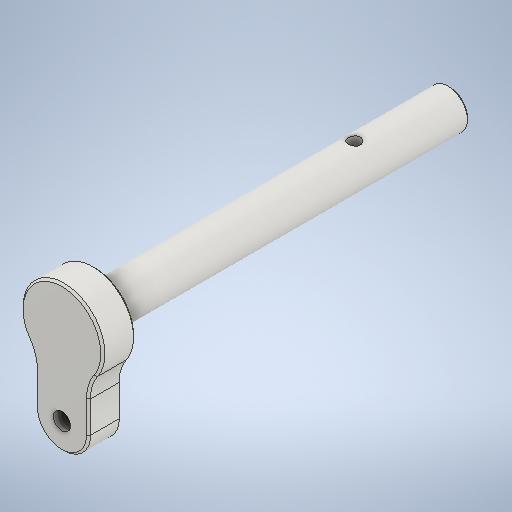
# Autodesk Inventor part: Crankshaft
Saved by Autodesk Inventor 2025.2 (Build 292293000, 293)
## iProperties
Created: 2025-06-12
Part Number: Crankshaft
Material: Steel AISI 1020 107 HR
Document SubType Name: Modeling
Designer: bless
Density: 7.87 g/cm^3
Appearance: Steel
Author: bless
Autodesk Inventor part; units mm, degrees
ref_plane "YZ Plane" through (0, 0, 0) normal (1, 0, 0) x (0, 1, 0)
ref_plane "XY Plane" through (0, 0, 0) normal (0, 0, 1) x (1, 0, 0)
sketch "Sketch1" plane through (0, 0, 0) normal (0, 0, 1) x (1, 0, 0)
  arc A0 (8.2491, -5.6527) -> (-8.2509, -5.65) centre (0, 0) ccw
  arc A1 (-6.5018, -19) -> (6.4982, -19) centre (-0.0018, -19) ccw
  circle A2 centre (0, 0) radius 4.75
  line L0 (-6.5018, -19) -> (-6.5018, -11.3)
  line L1 (6.4982, -19) -> (6.4982, -11.3053)
  arc A3 (-6.5018, -11.3) -> (-8.2509, -5.65) centre (-16.5018, -11.3) ccw
  arc A4 (8.2491, -5.6527) -> (6.4982, -11.3053) centre (16.4982, -11.3053) ccw
  point P0 (-6.5018, -7.5978)
  point P1 (6.4982, -7.6009)
  point P2 (-6.9491, -8.3427)
  dimension "d0" = 20
  dimension "d1" = 9.5
  dimension "d2" = 13
  dimension "d3" = 19
  dimension "d4" = 10
  dimension "d6" = 7.7
  constraints: 11 point on circle, 6 tangent, 5 centre point, 4 end point, 2 coincident, 2 point on line, 1 equal radius, 1 parallel, 1 vertical
  measures "d0" diameter of A0
  measures "d1" diameter of A2
  measures "d2" diameter of A1
  measures "d3" distance of A1.centre point (0, 0)
  measures "d4" radius of A3
  measures "d6" vertical distance of L0.end A1.centre
extrude "Extrusion1" add sketch "Sketch1" along normal blind 8
sketch "Sketch2" plane through (0, 0, 8) normal (0, 0, 1) x (1, 0, 0)
  arc A0 (-6.5018, -19) -> (6.4982, -19) centre (-0.0018, -19) ccw projected
hole "Hole1" at (-0.0018, -19, 8) direction (0, 0, -1) diameter 4.134 end through all thread size "M5x0.8" class "6H" standard "ANSI Metric M Profile"
sketch "Sketch3" plane through (0, 0, 8) normal (0, 0, 1) x (1, 0, 0)
  circle A0 centre (0, 0) radius 4.75 projected
  circle A1 centre (0, 0) radius 4.75
  constraints: 1 centre point, 1 coincident, 1 concentric
extrude "Extrusion2" add sketch "Sketch3" against normal blind 95
chamfer "Chamfer1" distance 0.5 angle 45 13 edges at (0.0016, 10, 8) (-6.9491, -8.3427, 8) (-6.5018, -15.15, 8) (-0.0018, -25.5, 8) (6.4982, -15.1527, 8) (6.9459, -8.3465, 8) (-4.75, 0, -87) (-0.0018, -25.5, 0) (6.4982, -15.1527, 0) (6.9459, -8.3465, 0) (0.0016, 10, 0) (-6.9491, -8.3427, 0) (-6.5018, -15.15, 0)
ref_plane "Work Plane1" through (0, 4.75, 0) normal (0, 1, 0) x (-1, 0, 0)
sketch "Sketch4" plane through (0, 4.75, 0) normal (0, 1, 0) x (-1, 0, 0)
  circle A0 centre (0, -63.5) radius 1.5
  line L0 (-4.75, -87) -> (4.75, -87) projected
  point P0 (0, 0)
  point P1 (0, -87)
  dimension "d22" = 3
  dimension "d23" = 23.5
  constraints: 1 centre point, 1 midpoint, 1 vertical alignment
  measures "d22" diameter of A0
  measures "d23" distance from line of L0 A0.centre
extrude "Extrusion3" cut sketch "Sketch4" against normal through all
body "Solid1"
